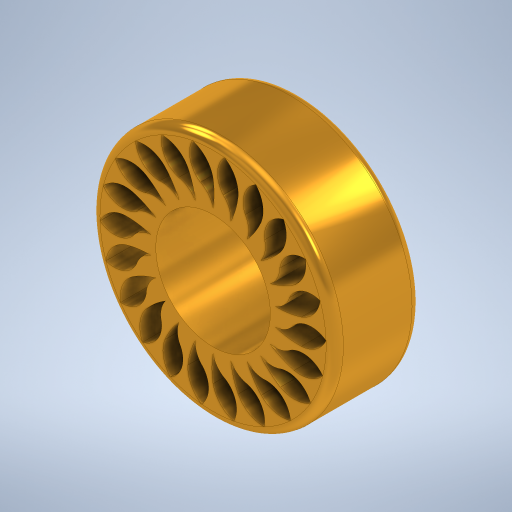
# Autodesk Inventor part: Idea2
Saved by Autodesk Inventor 2024.2 (Build 282272000, 272)
## iProperties
Created: 2025-06-20
Part Number: Idea2
Material: Generic
Document SubType Name: Modeling
Designer: Admin
Density: 1 g/cm^3
Appearance: Metal 1800F Hot
Author: Admin
Autodesk Inventor part; units mm, degrees
ref_plane "YZ Plane" through (0, 0, 0) normal (1, 0, 0) x (0, 1, 0)
ref_plane "XZ Plane" through (0, 0, 0) normal (0, 1, 0) x (-1, 0, 0)
ref_plane "XY Plane" through (0, 0, 0) normal (0, 0, 1) x (1, 0, 0)
sketch "Sketch1" plane through (0, 0, 0) normal (0, 0, 1) x (1, 0, 0)
  circle A0 centre (0, 0) radius 42.5
  circle A1 centre (0, 0) radius 20
  circle A2 centre (0, 0) radius 22 construction
  circle A3 centre (0, 0) radius 39.5 construction
  arc A4 (-7.2171, 38.8351) -> (-4.4005, 27.6363) centre (0.3428, 34.7829) ccw
  arc A5 (0, 22) -> (-4.4005, 27.6363) centre (-8.1056, 20.2077) ccw
  arc A6 (0, 31.1298) -> (-7.2171, 38.8351) centre (-9.9646, 29.029) ccw
  arc A7 (0, 22) -> (0, 31.1298) centre (-26.9361, 26.5649) ccw
  arc A8 (-8.7703, 29.8689) -> (-17.8659, 35.2287) centre (-17.7394, 25.0458) ccw
  arc A9 (-17.8659, 35.2287) -> (-12.0083, 25.2771) centre (-9.4706, 33.4705) ccw
  arc A10 (-6.1981, 21.1088) -> (-12.0083, 25.2771) centre (-13.4704, 17.1055) ccw
  arc A11 (-6.1981, 21.1088) -> (-8.7703, 29.8689) centre (-33.3292, 17.9001) ccw
  arc A12 (-16.8301, 26.1881) -> (-27.0673, 28.7683) centre (-24.0771, 19.0335) ccw
  arc A13 (-27.0673, 28.7683) -> (-18.6432, 20.8701) centre (-18.5167, 29.4466) ccw
  arc A14 (-11.8941, 18.5076) -> (-18.6432, 20.8701) centre (-17.7439, 12.6176) ccw
  arc A15 (-11.8941, 18.5076) -> (-16.8301, 26.1881) centre (-37.0222, 7.7851) ccw
  arc A16 (-23.5264, 20.3857) -> (-34.0758, 19.9772) centre (-28.4641, 11.4792) ccw
  arc A17 (-34.0758, 19.9772) -> (-23.7678, 14.7723) centre (-26.0627, 23.037) ccw
  arc A18 (-16.6265, 14.4069) -> (-23.7678, 14.7723) centre (-20.58, 7.1074) ccw
  arc A19 (-16.6265, 14.4069) -> (-23.5264, 20.3857) centre (-37.7158, -2.9606) ccw
  arc A20 (-28.3167, 12.9318) -> (-38.3237, 9.5678) centre (-30.5452, 2.995) ccw
  arc A21 (-38.3237, 9.5678) -> (-26.9669, 7.4777) centre (-31.4973, 14.7612) ccw
  arc A22 (-20.0119, 9.1391) -> (-26.9669, 7.4777) centre (-21.7487, 1.0215) ccw
  arc A23 (-20.0119, 9.1391) -> (-28.3167, 12.9318) centre (-35.354, -13.4665) ccw
  arc A24 (-30.813, 4.4302) -> (-39.4669, -1.6168) centre (-30.1517, -5.7319) ccw
  arc A25 (-39.4669, -1.6168) -> (-27.9813, -0.4226) centre (-34.3801, 5.2894) ccw
  arc A26 (-21.7761, 3.1309) -> (-27.9813, -0.4226) centre (-21.1555, -5.1472) ccw
  arc A27 (-21.7761, 3.1309) -> (-30.813, 4.4302) centre (-30.1279, -22.8813) ccw
  arc A28 (-30.813, -4.4302) -> (-37.4127, -12.6705) centre (-27.3155, -13.9945) ccw
  arc A29 (-37.4127, -12.6705) -> (-26.7288, -8.2887) centre (-34.4777, -4.6108) ccw
  arc A30 (-21.7761, -3.1309) -> (-26.7288, -8.2887) centre (-18.8484, -10.8989) ccw
  arc A31 (-21.7761, -3.1309) -> (-30.813, -4.4302) centre (-22.4611, -30.4425) ccw
  arc A32 (-28.3167, -12.9318) -> (-32.3275, -22.6976) centre (-22.2663, -21.1232) ccw
  arc A33 (-32.3275, -22.6976) -> (-23.3109, -15.4833) centre (-31.7821, -14.1375) ccw
  arc A34 (-20.0119, -9.1391) -> (-23.3109, -15.4833) centre (-15.0144, -15.7677) ccw
  arc A35 (-20.0119, -9.1391) -> (-28.3167, -12.9318) centre (-12.9746, -35.5374) ccw
  arc A36 (-23.5264, -20.3857) -> (-24.6234, -30.8859) centre (-15.4132, -26.5407) ccw
  arc A37 (-24.6234, -30.8859) -> (-18.0045, -21.4236) centre (-26.5117, -22.5189) ccw
  arc A38 (-16.6265, -14.4069) -> (-18.0045, -21.4236) centre (-9.9639, -19.359) ccw
  arc A39 (-16.6265, -14.4069) -> (-23.5264, -20.3857) centre (-2.437, -37.7533) ccw
  arc A40 (-16.8301, -26.1881) -> (-14.9244, -36.572) centre (-7.3115, -29.8081) ccw
  arc A41 (-14.9244, -36.572) -> (-11.2394, -25.6282) centre (-19.0934, -29.0759) ccw
  arc A42 (-11.8941, -18.5076) -> (-11.2394, -25.6282) centre (-4.1063, -21.382) ccw
  arc A43 (-11.8941, -18.5076) -> (-16.8301, -26.1881) centre (8.298, -36.9106) ccw
  arc A44 (-8.7703, -29.8689) -> (-4.0163, -39.2953) centre (1.3826, -30.6605) ccw
  arc A45 (-4.0163, -39.2953) -> (-3.5638, -27.7566) centre (-10.1284, -33.2774) ccw
  arc A46 (-6.1981, -21.1088) -> (-3.5638, -27.7566) centre (2.0841, -21.6727) ccw
  arc A47 (-6.1981, -21.1088) -> (-8.7703, -29.8689) centre (18.3608, -33.0776) ccw
  arc A48 (0, -31.1298) -> (7.2171, -38.8351) centre (9.9646, -29.029) ccw
  arc A49 (7.2171, -38.8351) -> (4.4005, -27.6363) centre (-0.3428, -34.7829) ccw
  arc A50 (0, -22) -> (4.4005, -27.6363) centre (8.1056, -20.2077) ccw
  arc A51 (0, -22) -> (0, -31.1298) centre (26.9361, -26.5649) ccw
  arc A52 (8.7703, -29.8689) -> (17.8659, -35.2287) centre (17.7394, -25.0458) ccw
  arc A53 (17.8659, -35.2287) -> (12.0083, -25.2771) centre (9.4706, -33.4705) ccw
  arc A54 (6.1981, -21.1088) -> (12.0083, -25.2771) centre (13.4704, -17.1055) ccw
  arc A55 (6.1981, -21.1088) -> (8.7703, -29.8689) centre (33.3292, -17.9001) ccw
  arc A56 (16.8301, -26.1881) -> (27.0673, -28.7683) centre (24.0771, -19.0335) ccw
  arc A57 (27.0673, -28.7683) -> (18.6432, -20.8701) centre (18.5167, -29.4466) ccw
  arc A58 (11.8941, -18.5076) -> (18.6432, -20.8701) centre (17.7439, -12.6176) ccw
  arc A59 (11.8941, -18.5076) -> (16.8301, -26.1881) centre (37.0222, -7.7851) ccw
  arc A60 (23.5264, -20.3857) -> (34.0758, -19.9772) centre (28.4641, -11.4792) ccw
  arc A61 (34.0758, -19.9772) -> (23.7678, -14.7723) centre (26.0627, -23.037) ccw
  arc A62 (16.6265, -14.4069) -> (23.7678, -14.7723) centre (20.58, -7.1074) ccw
  arc A63 (16.6265, -14.4069) -> (23.5264, -20.3857) centre (37.7158, 2.9606) ccw
  arc A64 (28.3167, -12.9318) -> (38.3237, -9.5678) centre (30.5452, -2.995) ccw
  arc A65 (38.3237, -9.5678) -> (26.9669, -7.4777) centre (31.4973, -14.7612) ccw
  arc A66 (20.0119, -9.1391) -> (26.9669, -7.4777) centre (21.7487, -1.0215) ccw
  arc A67 (20.0119, -9.1391) -> (28.3167, -12.9318) centre (35.354, 13.4665) ccw
  arc A68 (30.813, -4.4302) -> (39.4669, 1.6168) centre (30.1517, 5.7319) ccw
  arc A69 (39.4669, 1.6168) -> (27.9813, 0.4226) centre (34.3801, -5.2894) ccw
  arc A70 (21.7761, -3.1309) -> (27.9813, 0.4226) centre (21.1555, 5.1472) ccw
  arc A71 (21.7761, -3.1309) -> (30.813, -4.4302) centre (30.1279, 22.8813) ccw
  arc A72 (30.813, 4.4302) -> (37.4127, 12.6705) centre (27.3155, 13.9945) ccw
  arc A73 (37.4127, 12.6705) -> (26.7288, 8.2887) centre (34.4777, 4.6108) ccw
  arc A74 (21.7761, 3.1309) -> (26.7288, 8.2887) centre (18.8484, 10.8989) ccw
  arc A75 (21.7761, 3.1309) -> (30.813, 4.4302) centre (22.4611, 30.4425) ccw
  arc A76 (28.3167, 12.9318) -> (32.3275, 22.6976) centre (22.2663, 21.1232) ccw
  arc A77 (32.3275, 22.6976) -> (23.3109, 15.4833) centre (31.7821, 14.1375) ccw
  arc A78 (20.0119, 9.1391) -> (23.3109, 15.4833) centre (15.0144, 15.7677) ccw
  arc A79 (20.0119, 9.1391) -> (28.3167, 12.9318) centre (12.9746, 35.5374) ccw
  arc A80 (23.5264, 20.3857) -> (24.6234, 30.8859) centre (15.4132, 26.5407) ccw
  arc A81 (24.6234, 30.8859) -> (18.0045, 21.4236) centre (26.5117, 22.5189) ccw
  arc A82 (16.6265, 14.4069) -> (18.0045, 21.4236) centre (9.9639, 19.359) ccw
  arc A83 (16.6265, 14.4069) -> (23.5264, 20.3857) centre (2.437, 37.7533) ccw
  arc A84 (16.8301, 26.1881) -> (14.9244, 36.572) centre (7.3115, 29.8081) ccw
  arc A85 (14.9244, 36.572) -> (11.2394, 25.6282) centre (19.0934, 29.0759) ccw
  arc A86 (11.8941, 18.5076) -> (11.2394, 25.6282) centre (4.1063, 21.382) ccw
  arc A87 (11.8941, 18.5076) -> (16.8301, 26.1881) centre (-8.298, 36.9106) ccw
  arc A88 (8.7703, 29.8689) -> (4.0163, 39.2953) centre (-1.3826, 30.6605) ccw
  arc A89 (4.0163, 39.2953) -> (3.5638, 27.7566) centre (10.1284, 33.2774) ccw
  arc A90 (6.1981, 21.1088) -> (3.5638, 27.7566) centre (-2.0841, 21.6727) ccw
  arc A91 (6.1981, 21.1088) -> (8.7703, 29.8689) centre (-18.3608, 33.0776) ccw
  point P0 (3.5638, 27.7566)
  point P1 (27.9813, 0.4226)
  point P2 (26.9669, -7.4777)
  point P3 (18.6432, -20.8701)
  point P4 (4.4005, -27.6363)
  point P5 (-3.5638, -27.7566)
  point P6 (-23.3109, -15.4833)
  point P7 (-27.9813, -0.4226)
  point P8 (-26.9669, 7.4777)
  point P9 (-23.7678, 14.7723)
  point P10 (-18.6432, 20.8701)
  point P11 (-12.0083, 25.2771)
  dimension "d0" = 85
  dimension "d1" = 40
  dimension "d2" = 2
  dimension "d3" = 3
  dimension "d6" = 360
  constraints: 176 point on circle, 90 centre point, 4 coincident, 1 vertical alignment, 292 other
  measures "d0" diameter of A0
  measures "d1" diameter of A1
extrude "Extrusion1" add sketch "Sketch1" along normal blind 30
fillet "Fillet1" radius 3 2 edges at (-42.5, 0, 30) (-42.5, 0, 0)
body "Solid1"
